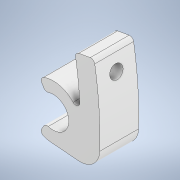
# Autodesk Inventor part: TH22_3DP_cover_fixer_sn
Saved by Autodesk Inventor 2022 (Build 260153000, 153)
## iProperties
Created: 2022-02-09
Part Number: TH22_3DP_cover_fixer_sn
Material: ABS プラスチック
Document SubType Name: Modeling
Designer: 中島 青蔵
Density: 1.06 g/cm^3
Appearance: 滑らか - 白
Author: 中島 青蔵
Autodesk Inventor part; units mm, degrees
ref_plane "YZ Plane" through (0, 0, 0) normal (1, 0, 0) x (0, 1, 0)
ref_plane "XZ Plane" through (0, 0, 0) normal (0, 1, 0) x (-1, 0, 0)
sketch "スケッチ1" plane through (0, 0, 0) normal (0, 0, 1) x (1, 0, 0)
  circle A0 centre (0, 0) radius 98.5
  circle A1 centre (0, 0) radius 86.5
  circle A2 centre (86.5, 0) radius 4
  circle A3 centre (86.5, 0) radius 7
  line L0 (0, 0) -> (98.5, 0)
  circle A4 centre (0, 0) radius 93.5
  line L1 (0, 0) -> (97.003564, 17.104346)
  line L2 (0, 0) -> (98.17694, -7.971098)
  line L3 (86.5, 0) -> (83, 6.062178)
  line L4 (86.5, 0) -> (83, -6.062178)
  line L5 (97.746748, 12.158256) -> (0, 0)
  point P0 (84.5, -3.464102)
  point P1 (83, -6.062178)
  point P2 (86.216763, -6.994267)
  point P3 (86.216298, -7)
  point P4 (92.079525, 16.236105)
  point P5 (93.5, 0)
  point P6 (84.5, 3.464102)
  dimension "d1" = 173
  dimension "d3" = 14
  dimension "d0" = 197
  dimension "d2" = 8
  dimension "d4" = 187
  dimension "d5" = 10
  dimension "d6" = 60
  dimension "d11" = 5
  dimension "d20" = 7.09
  constraints: 12 end point, 4 point on circle, 3 centre point, 3 coincident, 1 horizontal, 1 point on line, 1 symmetric about line, 7 other
  measures "d0" diameter of A0
  measures "d2" diameter of A2
  measures "d4" diameter of A4
  measures "d5" angle of L0 L1
  measures "d6" angle of L0 L3
  measures "d11" distance from line of L1 L5.start
sketch "スケッチ1 outline for 押し出し1" plane through (0, 0, 0) normal (0, 0, 1) x (1, 0, 0)
  arc A0 (84.5, 3.464102) -> (84.5, -3.464102) centre (86.5, 0) cw
  line L0 (83, 6.062178) -> (84.5, 3.464102)
  arc A1 (93.5, 0) -> (83, 6.062178) centre (86.5, 0) ccw
  arc A2 (92.079525, 16.236105) -> (93.5, 0) centre (0, 0) cw
  line L1 (97.003564, 17.104346) -> (92.079525, 16.236105)
  arc A3 (98.17694, -7.971098) -> (97.003564, 17.104346) centre (0, 0) ccw
  line L2 (86.216298, -7) -> (98.17694, -7.971098)
  arc A4 (86.216763, -6.994267) -> (86.216298, -7) centre (-0.000023, 0.000002) cw
  arc A5 (83, -6.062178) -> (86.216763, -6.994267) centre (86.5, 0) ccw
  line L3 (84.5, -3.464102) -> (83, -6.062178)
extrude "押し出し1" add sketch "スケッチ1 outline for 押し出し1" along normal blind 10
ref_plane "作業平面1" through (97.746748, 12.158256, 0) normal (0.9923528, 0.1234341, 0) x (-0.1234341, 0.9923528, 0)
sketch "スケッチ2" plane through (97.746748, 12.158256, 0) normal (0.9923528, 0.1234341, 0) x (-0.1234341, 0.9923528, 0)
  line L0 (5, 10) -> (-20.028521, 10)
  point P0 (0, 0)
  point P1 (0, 5)
  dimension "d12" = 5
  measures "d12" distance from line of L0 point (0, 5)
hole "穴1" at (97.746748, 12.158256, 5) direction (-0.9923528, -0.1234341, 0) diameter 3.4 end through all
fillet "フィレット1" radius 1 7 edges at (83, -6.0622, 5) (84.5, -3.4641, 5) (84.5, 3.4641, 5) (83, 6.0622, 5) (93.5, 0, 5) (92.0795, 16.2361, 5) (97.0036, 17.1043, 5)
fillet "フィレット2" radius 5 1 edges at (98.1769, -7.9711, 5)
